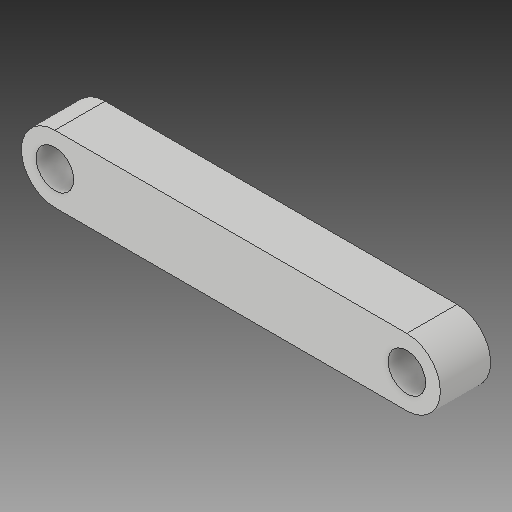
# Autodesk Inventor part: MassiveToe2
Saved by Autodesk Inventor 2017 (Build 210142000, 142)
## iProperties
Created: 2020-09-06
Part Number: MassiveToe2
Material: Generic
Document SubType Name: Modeling
Designer: agustin
Density: 1 g/cm^3
Appearance: Default
Author: agustin
Autodesk Inventor part; units mm, degrees
ref_plane "YZ Plane" through (0, 0, 0) normal (1, 0, 0) x (0, 1, 0)
ref_plane "XZ Plane" through (0, 0, 0) normal (0, 1, 0) x (-1, 0, 0)
ref_plane "XY Plane" through (0, 0, 0) normal (0, 0, 1) x (1, 0, 0)
sketch "Sketch1" plane through (0, 0, 0) normal (0, 0, 1) x (1, 0, 0)
  circle A0 centre (21, 0) radius 2.25 projected
  circle A1 centre (-21, 0) radius 2.25 projected
  line L0 (21, 0) -> (-21, 0) construction
  line L1 (21, 4) -> (-21, 4)
  line L2 (-21, -4) -> (21, -4)
  arc A2 (21, -4) -> (21, 4) centre (21, 0) ccw
  arc A3 (-21, 4) -> (-21, -4) centre (-21, 0) ccw
  point P0 (0, 0)
  point P1 (0, 0)
  dimension "d0" = 8
  constraints: 8 end point, 4 point on circle, 4 tangent, 2 centre point, 1 horizontal, 1 midpoint, 1 parallel
  measures "d0" diameter of A3
extrude "Extrusion1" add sketch "Sketch1" along normal blind 6
scale "Scale1" factors (0.5, 0.5, 0.5) then translate (0, -2, 3) bodies 1
body "Solid1"
